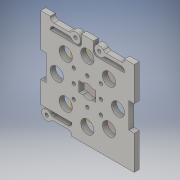
# Autodesk Inventor part: Bottom
Saved by Autodesk Inventor 2016 (Build 200138000, 138)
## iProperties
Created: 2015-06-30
Part Number: Bottom
Material: Generic
Document SubType Name: Modeling
Designer: Rodrigo
Density: 1 g/cm^3
Appearance: Default
Author: Rodrigo
Autodesk Inventor part; units mm, degrees
ref_plane "YZ Plane" through (0, 0, 0) normal (1, 0, 0) x (0, 1, 0)
ref_plane "XZ Plane" through (0, 0, 0) normal (0, 1, 0) x (-1, 0, 0)
ref_plane "XY Plane" through (0, 0, 0) normal (0, 0, 1) x (1, 0, 0)
ref_plane "Work Plane1" through (0, 0, 0) normal (0, 0, 1) x (1, 0, 0)
sketch "Sketch1" plane through (0, 0, 0) normal (0, 0, 1) x (1, 0, 0)
  circle A0 centre (6.5, 20.75) radius 1
  circle A1 centre (6.5, 4.75) radius 1
  circle A2 centre (22.5, 20.75) radius 1
  circle A3 centre (22.5, 4.75) radius 1
  line L0 (-13, -14.75) -> (42, -14.75)
  line L1 (42, -14.75) -> (42, 40.25)
  line L2 (42, 40.25) -> (-13, 40.25)
  line L3 (-13, 40.25) -> (-13, -14.75)
  line L4 (-13, -14.75) -> (42, 40.25) construction
  line L5 (42, -14.75) -> (-13, 40.25) construction
  circle A4 centre (22.5, 12.75) radius 1 projected
  circle A5 centre (14.5, 20.75) radius 1 projected
  circle A6 centre (14.5, 4.75) radius 1 projected
  circle A7 centre (6.5, 12.75) radius 1 projected
  line L6 (19.5, 15.75) -> (19.5, 9.75)
  line L7 (17.1458, 15.75) -> (19.5, 15.75)
  arc A8 (17.1458, 15.75) -> (11.8542, 15.75) centre (14.5, 12.75) ccw
  line L8 (9.5, 15.75) -> (11.8542, 15.75)
  line L9 (9.5, 9.75) -> (9.5, 15.75)
  line L10 (11.8542, 9.75) -> (9.5, 9.75)
  arc A9 (11.8542, 9.75) -> (17.1458, 9.75) centre (14.5, 12.75) ccw
  line L11 (19.5, 9.75) -> (17.1458, 9.75)
  point P0 (0, 0)
  dimension "d0" = 55
  dimension "d1" = 55
  dimension "d95" = 2
  dimension "d96" = 2
  dimension "d97" = 2
  dimension "d98" = 2
  constraints: 24 end point, 6 centre point, 4 point on circle, 2 midpoint, 2 parallel, 1 horizontal, 1 perpendicular
  measures "d0" distance of L2.end L1.end
  measures "d1" distance of L1.end L0.end
  measures "d95" diameter of A0
  measures "d96" diameter of A2
  measures "d97" diameter of A3
  measures "d98" diameter of A1
extrude "Extrusion3" add sketch "Sketch1" along normal blind 3
sketch "Sketch4" plane through (0, 0, 3) normal (0, 0, 1) x (1, 0, 0)
  line L0 (42, 40.25) -> (-13, 40.25) construction
  line L1 (14.5, 40.25) -> (14.5, 12.75) construction
  line L2 (-13, -14.75) -> (42, -14.75) construction
  line L3 (-13, 40.25) -> (-13, -14.75) construction
  line L4 (-13, 12.75) -> (14.5, 12.75) construction
  circle A0 centre (14.5, 30.75) radius 3.895
  circle A1 centre (1.7721, 25.4779) radius 3.895
  circle A2 centre (-3.5, 12.75) radius 3.895
  circle A3 centre (1.7721, 0.0221) radius 3.895
  circle A4 centre (14.5, -5.25) radius 3.895
  circle A5 centre (27.2279, 0.0221) radius 3.895
  circle A6 centre (32.5, 12.75) radius 3.895
  circle A7 centre (27.2279, 25.4779) radius 3.895
  arc A8 (4.6716, 35.75) -> (4.6716, 37.75) centre (7.5, 36.75) ccw
  line L5 (42, 40.25) -> (-13, 40.25)
  line L6 (7.5, 36.75) -> (-13, 36.75) construction
  line L7 (4.6716, 37.75) -> (-7.3284, 37.75)
  line L8 (4.6716, 35.75) -> (-7.3284, 35.75)
  line L9 (-7.3284, 37.75) -> (-7.3284, 40.25)
  line L10 (10.9716, 40.25) -> (-7.3284, 40.25)
  line L11 (-7.3284, 35.75) -> (-7.3284, 33.25)
  line L12 (-7.3284, 33.25) -> (10.9716, 33.25)
  line L13 (10.9716, 40.25) -> (10.9716, 33.25)
  arc A9 (24.3284, 37.75) -> (24.3284, 35.75) centre (21.5, 36.75) ccw
  line L14 (24.3284, 37.75) -> (36.3284, 37.75)
  line L15 (24.3284, 35.75) -> (36.3284, 35.75)
  line L16 (36.3284, 37.75) -> (36.3284, 40.25)
  line L17 (18.0284, 40.25) -> (36.3284, 40.25)
  line L18 (36.3284, 35.75) -> (36.3284, 33.25)
  line L19 (36.3284, 33.25) -> (18.0284, 33.25)
  line L20 (18.0284, 40.25) -> (18.0284, 33.25)
  arc A10 (-6.6716, -10.25) -> (-6.6716, -12.25) centre (-9.5, -11.25) ccw
  line L21 (-9.5, -11.25) -> (8.4531, -11.25) construction
  line L22 (-6.6716, -10.25) -> (5.3284, -10.25)
  line L23 (-6.6716, -12.25) -> (5.3284, -12.25)
  line L24 (5.3284, -12.25) -> (5.3284, -14.75)
  line L25 (5.3284, -10.25) -> (5.3284, -7.75)
  line L26 (5.3284, -7.75) -> (-13, -7.75)
  line L27 (-13, -14.75) -> (-13, -7.75)
  line L28 (-13, -14.75) -> (5.3284, -14.75)
  point P0 (0, 0)
  dimension "d24" = 7.79
  dimension "d25" = 18
  dimension "d28" = 360
  dimension "d63" = 6
  dimension "d64" = 7
  dimension "d65" = 12
  dimension "d66" = 18.3
  dimension "d67" = 2.5
  dimension "d68" = 3.5
  dimension "d71" = 1
  dimension "d74" = 6
  dimension "d75" = 3.5
  dimension "d76" = 3.5
  dimension "d77" = 12
  dimension "d78" = 1
  dimension "d79" = 2.5
  constraints: 58 end point, 14 symmetric about line, 11 centre point, 6 point on circle, 6 point on line, 5 perpendicular, 4 horizontal, 3 coincident, 3 collinear, 3 vertical, 2 midpoint, 18 other
  measures "d24" diameter of A0
  measures "d25" distance of L1.end A0.centre
  measures "d63" diameter of A8
  measures "d64" distance from line of L1 L6.start
  measures "d65" distance of L7.start L7.end
  measures "d66" distance of L10.start L9.end
  measures "d67" distance between parallel lines of L12 L8
  measures "d68" distance from line of L10 L6.start
  measures "d71" distance between parallel lines of L7 L6
  measures "d74" diameter of A10
  measures "d75" distance from line of L21.start L2
  measures "d76" distance from line of L3 L21.start
  measures "d77" distance of L22.start L22.end
  measures "d78" distance between parallel lines of L22 L21
  measures "d79" distance of L22.end L25.end
extrude "Extrusion2" cut sketch "Sketch4" against normal through all
hole "Hole4" at (7.5, 36.75, 3) at (21.5, 36.75, 3) at (-9.5, -11.25, 3) direction (0, 0, -1) diameter 2 end through all
fillet "Fillet3" radius 2 14 edges at (-7.3284, 35.75, 1.5) (-7.3284, 37.75, 1.5) (4.6716, 37.75, 1.5) (4.6716, 35.75, 1.5) (10.9716, 33.25, 1.5) (24.3284, 37.75, 1.5) (24.3284, 35.75, 1.5) (36.3284, 37.75, 1.5) (36.3284, 35.75, 1.5) (18.0284, 33.25, 1.5) (5.3284, -10.25, 1.5) (5.3284, -12.25, 1.5) (-6.6716, -10.25, 1.5) (-6.6716, -12.25, 1.5)
sketch "Sketch6" plane through (0, 0, 3) normal (0, 0, 1) x (1, 0, 0)
  line L0 (38.85, 20.3) -> (42, 20.3)
  line L1 (42, 20.3) -> (42, 5.2)
  line L2 (42, 5.2) -> (38.85, 5.2)
  line L3 (38.85, 5.2) -> (38.85, 20.3)
  line L4 (42, -14.75) -> (42, 40.25) projected
  line L5 (18.0284, 40.25) -> (10.9716, 40.25) construction
  line L6 (14.5, 40.25) -> (14.5, -14.75) construction
  line L7 (5.3284, -14.75) -> (42, -14.75) construction
  line L8 (-9.85, 20.3) -> (-13, 20.3)
  line L9 (-13, 20.3) -> (-13, 5.2)
  line L10 (-13, 5.2) -> (-9.85, 5.2)
  line L11 (-9.85, 5.2) -> (-9.85, 20.3)
  line L12 (-13, -14.75) -> (-13, 40.25)
  point P0 (0, 0)
  point P1 (42, 12.75)
  point P2 (42, 12.75)
  point P3 (-13, 12.75)
  point P4 (-13, 12.75)
  dimension "d91" = 3.15
  dimension "d92" = 15.1
  constraints: 20 end point, 8 symmetric about line, 3 midpoint, 3 point on line, 2 parallel, 1 coincident, 1 horizontal, 1 perpendicular, 1 vertical
  measures "d91" distance of L1.end L2.end
  measures "d92" distance of L0.end L1.end
extrude "Extrusion4" cut sketch "Sketch6" against normal through all
equation "\"d38\" = d24"
body "Solid1"
body "Solid2"
